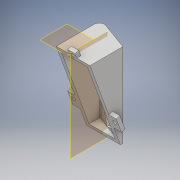
# Autodesk Inventor part: k2_t_l1a
Saved by Autodesk Inventor 2017 (Build 210142000, 142)
## iProperties
Created: 2017-02-10
Part Number: k2_t_l1a
Material: Generic
Document SubType Name: Modeling
Designer: herman
Density: 1 g/cm^3
Appearance: Default
Author: herman
Autodesk Inventor part; units mm, degrees
ref_plane "YZ Plane" through (0, 0, 0) normal (1, 0, 0) x (0, 1, 0)
ref_plane "XZ Plane" through (0, 0, 0) normal (0, 1, 0) x (-1, 0, 0)
ref_plane "XY Plane" through (0, 0, 0) normal (0, 0, 1) x (1, 0, 0)
ref_plane "Work Plane1" through (0, -11.6382, 33.3368) normal (0, 0, 1) x (1, 0, 0)
sketch "Sketch7" plane through (0, -11.6382, 33.3368) normal (0, 0, 1) x (1, 0, 0)
  line L0 (0, 15.5588) -> (27, 15.5588)
  line L1 (27, 15.5588) -> (27, 17.5588)
  line L2 (27, 17.5588) -> (0, 27.386)
  line L3 (0, 27.386) -> (0, 15.5588)
  line L4 (0, 15.5588) -> (27, 15.5588)
  point P0 (0, 11.6382)
  dimension "d20" = 2
  dimension "d21" = 110
  dimension "d76" = 27
  constraints: 10 end point, 1 collinear, 1 perpendicular, 1 vertical
  measures "d20" distance of L0.end L1.end
  measures "d21" angle of L2 L1
  measures "d76" distance of L0.start L0.end
extrude "Extrusion5" add sketch "Sketch7" against normal blind 67
sketch "Sketch8" plane through (0, 3.9206, 33.3368) normal (-1, 0, 0) x (0, 0, 1)
  line L0 (0, 0) -> (-67, 0) projected
  line L1 (-67, 0) -> (0, -24.386)
  line L2 (0, -24.386) -> (0, 0)
  point P0 (-33.3368, -3.9206)
  dimension "d27" = 20
  constraints: 4 end point, 1 vertical
  measures "d27" angle of L0 L1
extrude "Extrusion6" add sketch "Sketch8" against normal up to surface (27 mm away)
shell "Shell3" thickness 3 removed faces 1 at (9, -4.2081, -11.3299)
sketch "Sketch9" plane through (27, 5.9206, 33.3368) normal (0.3420201, 0.9396926, 0) x (0.9396926, -0.3420201, 0)
  line L0 (-21.711, 26.8228) -> (-7.711, 26.8228)
  line L1 (-7.711, 26.8228) -> (-7.711, 40.8228)
  line L2 (-7.711, 40.8228) -> (-21.711, 40.8228)
  line L3 (-21.711, 40.8228) -> (-21.711, 26.8228)
  line L4 (-7.711, 33.8228) -> (47.289, 33.8228) construction
  line L5 (-15.1557, 3.6455) -> (-2, 8.4338)
  line L6 (-2, 8.4338) -> (-6.7883, 21.5895)
  line L7 (-6.7883, 21.5895) -> (-19.944, 16.8012)
  line L8 (-19.944, 16.8012) -> (-15.1557, 3.6455)
  line L9 (-19.944, 50.8443) -> (-6.7883, 46.056)
  line L10 (-6.7883, 46.056) -> (-2, 59.2117)
  line L11 (-2, 59.2117) -> (-15.1557, 64)
  line L12 (-15.1557, 64) -> (-19.944, 50.8443)
  line L13 (0, 0) -> (0, 67) projected
  line L14 (-28.7328, 67) -> (0, 67) projected
  point P0 (-4.3941, 15.0117)
  point P1 (-4.3941, 52.6339)
  dimension "d31" = 14
  dimension "d32" = 55
  dimension "d35" = 20
  dimension "d39" = 20
  dimension "d41" = 2
  dimension "d42" = 3
  constraints: 26 end point, 3 equal length, 2 horizontal, 2 parallel, 1 midpoint, 1 perpendicular, 20 other
  measures "d31" distance of L1.end L2.end
  measures "d32" distance of L4.start L4.end
  measures "d41" distance from line of L13 L10.end
  measures "d42" distance from line of L14 L11.end
extrude "Extrusion7" cut sketch "Sketch9" against normal up to next
fillet "Fillet1" radius 4 1 edges at (0, 15.7478, -0.1632)
sketch "Sketch10" plane through (27, 5.9206, 33.3368) normal (1, 0, 0) x (0, 0, -1)
  line L0 (0, -26.386) -> (67, -2) projected
  line L1 (41.6283, -11.2345) -> (40.6022, -8.4155)
  line L2 (40.6022, -8.4155) -> (51.8786, -4.3112)
  line L3 (51.8786, -4.3112) -> (52.9046, -7.1303)
  point P0 (33.3368, -5.9206)
  dimension "d46" = 3
  dimension "d47" = 12
  dimension "d48" = 15
  constraints: 6 end point, 3 perpendicular, 2 point on line
  measures "d46" distance of L1.start L1.end
  measures "d47" distance of L1.end L2.end
  measures "d48" distance of L0.end L3.end
ref_plane "Work Plane2" through (13.5, 5.9206, 33.3368) normal (1, 0, 0) x (0, 0, -1)
extrude "Extrusion8" add sketch "Sketch10" along normal blind 6
sketch "Sketch11" plane through (27, -2.4949, -7.2655) normal (0, 0.9396926, 0.3420201) x (1, 0, 0)
  line L0 (0, 0) -> (6, 0) projected
  line L1 (6, 12) -> (6, 0) projected
  point P0 (-27, -5.974)
  point P1 (3, 5)
  dimension "d52" = 5
  dimension "d53" = 3
  measures "d52" distance from line of L0 point (3, 5)
  measures "d53" distance from line of L1 point (3, 5)
hole "Hole1" at (30, -0.7848, -11.9639) direction (0, -0.9396926, -0.3420201) diameter 3 end through all
mirror "Mirror2" about plane through (13.5, 5.9206, 33.3368) normal (1, 0, 0) of "Extrusion8", "Hole1"
sketch "Sketch12" plane through (0, 3.9206, -33.6632) normal (0, -0.9396926, -0.3420201) x (1, 0, 0)
  line L0 (3, 68.1074) -> (24, 68.1074) projected
  line L1 (10.5, 68.1074) -> (16.5, 68.1074)
  line L2 (16.5, 68.1074) -> (16.5, 75.063)
  line L3 (16.5, 75.063) -> (10.5, 75.063)
  line L4 (10.5, 75.063) -> (10.5, 68.1074)
  line L5 (27, 0) -> (0, 0) projected
  line L6 (27, 71.2999) -> (27, 27) projected
  point P0 (0, 32.974)
  dimension "d61" = 75.063
  dimension "d62" = 6
  dimension "d64" = 10.5
  constraints: 8 end point, 2 parallel, 1 horizontal, 1 perpendicular, 1 point on line
  measures "d61" distance between parallel lines of L5 L3
  measures "d62" distance of L2.end L3.end
  measures "d64" distance between parallel lines of L6 L2
extrude "Extrusion9" add sketch "Sketch12" against normal blind 3
sketch "Sketch13" plane through (0, 6.7397, -32.6372) normal (0, 0.9396926, 0.3420201) x (1, 0, 0)
  line L0 (10.5, -75.063) -> (16.5, -75.063) projected
  line L1 (16.5, -75.063) -> (16.5, -70.208) projected
  point P0 (0, -32.974)
  point P1 (13.5, -72.063)
  dimension "d67" = 3
  dimension "d68" = 3
  measures "d67" distance from line of L0 point (13.5, -72.063)
  measures "d68" distance from line of L1 point (13.5, -72.063)
hole "Hole2" at (13.5, -17.9073, 35.0799) direction (0, -0.9396926, -0.3420201) diameter 3 end through all
body "Solid2"
